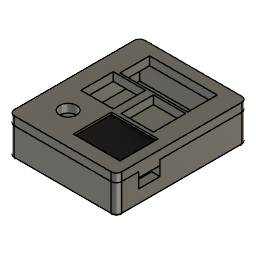
Hackpad case (Autodesk Fusion 360 design; units mm, degrees)
Autodesk Fusion 360 part; units mm, degrees
sketch "Sketch1" plane through (0, 0, 0) normal (0, 0, 1) x (1, 0, 0)
  line L0 (-43.0674, 74.3776) -> (-0.0674, 74.3776)
  line L1 (-0.0674, 74.3776) -> (-0.0674, 20.3776)
  line L2 (-0.0674, 20.3776) -> (-43.0674, 20.3776)
  line L3 (-43.0674, 20.3776) -> (-43.0674, 74.3776)
  line L4 (-0.0674, 20.3776) -> (-0.0674, 28.1436)
  line L5 (-0.0674, 26.9886) -> (3.8652, 26.9886)
  line L6 (-0.0674, 37.0541) -> (3.8652, 37.0541)
  line L7 (-47, 78.3102) -> (3.8652, 78.3102)
  line L8 (3.8652, 78.3102) -> (3.8652, 16.445)
  line L9 (3.8652, 16.445) -> (-47, 16.445)
  line L10 (-47, 16.445) -> (-47, 78.3102)
  dimension "d1" = 54
  dimension "d2" = 43
  constraint horizontal L0
  constraint vertical L1
  constraint horizontal L2
  constraint vertical L3
  constraint coincident L1 L4.end
  constraint coincident L1 L5.start
  constraint perpendicular L1 L5
  constraint coincident L1 L6.start
  constraint perpendicular L1 L6
  constraint horizontal L7
  constraint vertical L8
  constraint horizontal L9
  constraint vertical L10
  constraint coincident L5.end L8
  measures "d1" distance of L0.start L2.end
  measures "d2" distance of L0.start L0.end
extrude "Extrude1" add sketch "Sketch1" along normal blind 4 makes body 1
extrude "Extrude2" add sketch "Sketch1" along normal blind 13 contours L0 L1 L2 L3 L4 L5 L6 L7 L8 L9 L10 | L1 L4 L5 L6 L8 bodies 1
extrude "Extrude3" add sketch "Sketch1" along normal blind 14 contours L0 L1 L2 L3 L4 L5 L6 L7 L8 L9 L10 bodies 1
extrude "Extrude4" cut 1 faces at (2.5543, 33.6989, 13) along direction (0, 0, -1) blind 5 on bodies 1 bodies 1
fillet "Fillet1" radius 2.5 4 edges at (3.8652, 78.3102, 7) (-47, 78.3102, 7) (-47, 16.445, 7) (3.8652, 16.445, 7) on bodies 1
fillet "Fillet2" radius 1 8 edges at (3.1329, 17.1773, 0) (-21.5674, 16.445, 0) (-46.2678, 17.1773, 0) (-47, 47.3776, 0) (-46.2678, 77.578, 0) (-21.5674, 78.3102, 0) (3.1329, 77.578, 0) (3.8652, 47.3776, 0) on bodies 1
sketch "Sketch2" plane through (0, 0, 0) normal (0, 0, -1) x (1, 0, 0)
  arc A0 (2.8652, -18.945) -> (1.3652, -17.445) centre (1.3652, -18.945) ccw
  line L0 (1.3652, -17.445) -> (-44.5, -17.445)
  arc A1 (-44.5, -17.445) -> (-46, -18.945) centre (-44.5, -18.945) ccw
  line L1 (-46, -18.945) -> (-46, -75.8102)
  arc A2 (-46, -75.8102) -> (-44.5, -77.3102) centre (-44.5, -75.8102) ccw
  line L2 (-44.5, -77.3102) -> (1.3652, -77.3102)
  arc A3 (1.3652, -77.3102) -> (2.8652, -75.8102) centre (1.3652, -75.8102) ccw
  line L3 (2.8652, -75.8102) -> (2.8652, -18.945)
  circle A4 centre (-40, -25) radius 2.9748
  circle A5 centre (-31.25, -25) radius 2.9748
  circle A6 centre (-22.5, -25) radius 2.9748
  circle A7 centre (-13.75, -25) radius 2.9748
  circle A8 centre (-5, -25) radius 2.9748
  circle A9 centre (-40, -36.25) radius 2.9748
  circle A10 centre (-31.25, -36.25) radius 2.9748
  circle A11 centre (-22.5, -36.25) radius 2.9748
  circle A12 centre (-13.75, -36.25) radius 2.9748
  circle A13 centre (-5, -36.25) radius 2.9748
  circle A14 centre (-40, -47.5) radius 2.9748
  circle A15 centre (-31.25, -47.5) radius 2.9748
  circle A16 centre (-22.5, -47.5) radius 2.9748
  circle A17 centre (-13.75, -47.5) radius 2.9748
  circle A18 centre (-5, -47.5) radius 2.9748
  circle A19 centre (-40, -58.75) radius 2.9748
  circle A20 centre (-31.25, -58.75) radius 2.9748
  circle A21 centre (-22.5, -58.75) radius 2.9748
  circle A22 centre (-13.75, -58.75) radius 2.9748
  circle A23 centre (-5, -58.75) radius 2.9748
  circle A24 centre (-40, -70) radius 2.9748
  circle A25 centre (-31.25, -70) radius 2.9748
  circle A26 centre (-22.5, -70) radius 2.9748
  circle A27 centre (-13.75, -70) radius 2.9748
  circle A28 centre (-5, -70) radius 2.9748
  point P0 (-33, -25)
  point P1 (-26, -25)
  point P2 (-19, -25)
  point P3 (-12, -25)
  point P4 (-5, -25)
  point P5 (-40, -50)
  point P6 (-33, -50)
  point P7 (-26, -50)
  point P8 (-19, -50)
  point P9 (-12, -50)
  point P10 (-5, -50)
  point P11 (-40, -75)
  point P12 (-33, -75)
  point P13 (-26, -75)
  point P14 (-19, -75)
  point P15 (-12, -75)
  point P16 (-5, -75)
  dimension "d19" = 35
  dimension "d20" = -50
  dimension "d23" = 35
  dimension "d24" = -45
extrude "Extrude5" cut sketch "Sketch2" against normal blind 1 contours A4 | A5 | A6 | A7 | A9 | A10 | A11 | A12 | A13 | A14 | A15 | A16 | A17 | A18 | A19 | A20 | A21 | A22 | A23 | A25 | A26 | A27 | A28 bodies 1
extrude "Extrude6" cut sketch "Sketch2" against normal blind 1 contours A24 bodies 1
extrude "Extrude7" cut sketch "Sketch2" against normal blind 1 contours A8 bodies 1
sketch "Sketch3" plane through (0, 0, 14) normal (0, 0, 1) x (-1, 0, 0)
  arc A0 (-1.3652, -16.445) -> (-3.8652, -18.945) centre (-1.3652, -18.945) ccw
  line L0 (-3.8652, -18.945) -> (-3.8652, -26.9886)
  line L1 (-3.8652, -26.9886) -> (0.0674, -26.9886)
  line L2 (0.0674, -26.9886) -> (0.0674, -20.3776)
  line L3 (0.0674, -20.3776) -> (43.0674, -20.3776)
  line L4 (43.0674, -20.3776) -> (43.0674, -74.3776)
  line L5 (43.0674, -74.3776) -> (0.0674, -74.3776)
  line L6 (0.0674, -74.3776) -> (0.0674, -37.0541)
  line L7 (0.0674, -37.0541) -> (-3.8652, -37.0541)
  line L8 (-3.8652, -37.0541) -> (-3.8652, -75.8102)
  arc A1 (-3.8652, -75.8102) -> (-1.3652, -78.3102) centre (-1.3652, -75.8102) ccw
  line L9 (-1.3652, -78.3102) -> (44.5, -78.3102)
  arc A2 (44.5, -78.3102) -> (47, -75.8102) centre (44.5, -75.8102) ccw
  line L10 (47, -75.8102) -> (47, -18.945)
  arc A3 (47, -18.945) -> (44.5, -16.445) centre (44.5, -18.945) ccw
  line L11 (44.5, -16.445) -> (-1.3652, -16.445)
  line L12 (47.0064, -78.3102) -> (-3.8652, -78.3102)
  line L13 (-3.8652, -78.3102) -> (-3.8652, -16.4024)
  line L14 (-3.8652, -16.4024) -> (47.0064, -16.4024)
  line L15 (47.0064, -16.4024) -> (47.0064, -78.3102)
  constraint horizontal L12
  constraint vertical L13
  constraint horizontal L14
  constraint vertical L15
move_body "Move1" bodies 1 to x (1, 0, 0) y (0, 1, 0) z (0, 0, 1) at (0, -3, 0)
extrude "Extrude8" cut 1 faces at (2.5543, 30.6989, 8) along direction (0, 0, -1) blind 1 on bodies 1 bodies 1
sketch "Sketch4" plane through (0, 23.9886, 0) normal (0, 1, 0) x (-1, 0, 0)
  line L0 (0.0674, 7) -> (0.0674, 14)
  line L1 (0.0674, 14) -> (-3.8652, 14)
  line L2 (-3.8652, 14) -> (-3.8652, 7)
  line L3 (-3.8652, 7) -> (0.0674, 7)
sketch "Sketch5" plane through (0, 0, 14) normal (0, 0, 1) x (-1, 0, 0)
  arc A0 (-1.3652, -13.445) -> (-3.8652, -15.945) centre (-1.3652, -15.945) ccw
  line L0 (-3.8652, -15.945) -> (-3.8652, -23.9886)
  line L1 (-3.8652, -23.9886) -> (0.0674, -23.9886)
  line L2 (0.0674, -23.9886) -> (0.0674, -17.3776)
  line L3 (0.0674, -17.3776) -> (43.0674, -17.3776)
  line L4 (43.0674, -17.3776) -> (43.0674, -71.3776)
  line L5 (43.0674, -71.3776) -> (0.0674, -71.3776)
  line L6 (0.0674, -71.3776) -> (0.0674, -34.0541)
  line L7 (0.0674, -34.0541) -> (-3.8652, -34.0541)
  line L8 (-3.8652, -34.0541) -> (-3.8652, -72.8102)
  arc A1 (-3.8652, -72.8102) -> (-1.3652, -75.3102) centre (-1.3652, -72.8102) ccw
  line L9 (-1.3652, -75.3102) -> (44.5, -75.3102)
  arc A2 (44.5, -75.3102) -> (47, -72.8102) centre (44.5, -72.8102) ccw
  line L10 (47, -72.8102) -> (47, -15.945)
  arc A3 (47, -15.945) -> (44.5, -13.445) centre (44.5, -15.945) ccw
  line L11 (44.5, -13.445) -> (-1.3652, -13.445)
  line L12 (39.119, -54.9533) -> (23.8738, -54.9533)
  line L13 (23.8738, -54.9533) -> (23.8738, -39.7082)
  line L14 (23.8738, -39.7082) -> (39.119, -39.7082)
  line L15 (39.119, -39.7082) -> (39.119, -54.9533)
  line L16 (24.9964, -53.8308) -> (37.9964, -53.8308)
  line L17 (37.9964, -53.8308) -> (37.9964, -40.8308)
  line L18 (37.9964, -40.8308) -> (24.9964, -40.8308)
  line L19 (24.9964, -40.8308) -> (24.9964, -53.8308)
  line L20 (37.9964, -40.8308) -> (39.119, -39.7082)
  line L21 (24.9964, -53.8308) -> (23.8738, -54.9533)
  line L22 (39.119, -54.9533) -> (23.8738, -54.9533)
  line L23 (39.119, -39.7082) -> (39.119, -54.9533)
  line L24 (37.9964, -40.8308) -> (24.9964, -40.8308)
  line L25 (23.8738, -39.7082) -> (39.119, -39.7082)
  line L26 (37.9964, -40.8308) -> (39.119, -39.7082)
  line L27 (37.9964, -53.8308) -> (37.9964, -40.8308)
  line L28 (24.9964, -53.8308) -> (37.9964, -53.8308)
  line L29 (23.8738, -54.9533) -> (23.8738, -39.7082)
  line L30 (24.9964, -40.8308) -> (24.9964, -53.8308)
  line L31 (24.9964, -53.8308) -> (23.8738, -54.9533)
  line L32 (4.8738, -39.7082) -> (20.119, -39.7082)
  line L33 (4.8738, -54.9533) -> (4.8738, -39.7082)
  line L34 (5.9964, -53.8308) -> (18.9964, -53.8308)
  line L35 (5.9964, -40.8308) -> (5.9964, -53.8308)
  line L36 (18.9964, -40.8308) -> (5.9964, -40.8308)
  line L37 (20.119, -39.7082) -> (20.119, -54.9533)
  line L38 (20.119, -54.9533) -> (4.8738, -54.9533)
  line L39 (5.9964, -40.8308) -> (5.9964, -53.8308)
  line L40 (4.8738, -39.7082) -> (20.119, -39.7082)
  line L41 (20.119, -54.9533) -> (4.8738, -54.9533)
  line L42 (18.9964, -40.8308) -> (5.9964, -40.8308)
  line L43 (5.9964, -53.8308) -> (18.9964, -53.8308)
  line L44 (5.9964, -53.8308) -> (4.8738, -54.9533)
  line L45 (18.9964, -53.8308) -> (18.9964, -40.8308)
  line L46 (18.9964, -53.8308) -> (18.9964, -40.8308)
  line L47 (5.9964, -53.8308) -> (4.8738, -54.9533)
  line L48 (4.8738, -54.9533) -> (4.8738, -39.7082)
  line L49 (18.9964, -40.8308) -> (20.119, -39.7082)
  line L50 (18.9964, -40.8308) -> (20.119, -39.7082)
  line L51 (20.119, -39.7082) -> (20.119, -54.9533)
  line L52 (37, -70) -> (5, -70)
  line L53 (5, -70) -> (5, -56)
  line L54 (5, -56) -> (37, -56)
  line L55 (37, -56) -> (37, -70)
  line L56 (34, -32.5) -> (34, -24.5)
  circle A4 centre (34, -28.5) radius 4
  line L57 (23, -38) -> (1, -38)
  line L58 (1, -38) -> (1, -20.0095)
  line L59 (1, -20.0095) -> (23, -20.0095)
  line L60 (23, -20.0095) -> (23, -38)
  line L61 (-3.8652, -75.6763) -> (-3.8652, -13.0993)
  line L62 (-3.8652, -13.0993) -> (47, -13.0993)
  line L63 (47, -13.0993) -> (47, -75.6763)
  dimension "d33" = 13
  dimension "d34" = 13
  dimension "d35" = 13
  dimension "d36" = 13
  constraint horizontal L12
  constraint vertical L13
  constraint horizontal L14
  constraint vertical L15
  constraint horizontal L16
  constraint vertical L17
  constraint horizontal L18
  constraint vertical L19
  constraint equal L16 L19
  constraint equal L20 L21
  constraint parallel L20 L21
  constraint equal L12 L15
  constraint horizontal L22
  constraint vertical L29
  constraint horizontal L25
  constraint vertical L23
  constraint horizontal L28
  constraint vertical L27
  constraint horizontal L24
  constraint vertical L30
  constraint equal L28 L30
  constraint equal L26 L31
  constraint parallel L26 L31
  constraint equal L22 L23
  constraint horizontal L41
  constraint vertical L33
  constraint horizontal L40
  constraint vertical L37
  constraint horizontal L43
  constraint vertical L46
  constraint horizontal L36
  constraint vertical L35
  constraint equal L35 L43
  constraint equal L44 L50
  constraint parallel L44 L50
  constraint equal L37 L41
  constraint horizontal L38
  constraint vertical L48
  constraint horizontal L32
  constraint vertical L51
  constraint horizontal L34
  constraint vertical L45
  constraint horizontal L42
  constraint vertical L39
  constraint equal L34 L39
  constraint equal L47 L49
  constraint parallel L47 L49
  constraint equal L38 L51
  constraint horizontal L52
  constraint vertical L53
  constraint horizontal L54
  constraint vertical L55
  constraint vertical L56
  constraint horizontal L57
  constraint vertical L58
  constraint horizontal L59
  constraint vertical L60
  constraint vertical L61
  constraint horizontal L62
  constraint vertical L63
  measures "d33" distance of L16.end L17.end
  measures "d34" distance of L17.end L16.end
  measures "d35" distance of L36.start L34.end
  measures "d36" distance of L36.start L34.end
extrude "Extrude1'" add sketch "Sketch5" along normal blind 4 separate body contours A0 L0 L1 L2 L3 L4 L5 L6 L7 L8 A1 L9 A2 L10 A3 L11 L61 L63 | L1 L2 L3 L4 L5 L6 L7 L61 makes body 2 in component "Component"
sketch "Sketch6" plane through (0, 0, 14) normal (0, 0, -1) x (1, 0, 0)
  line L0 (-20.119, -39.7082) -> (-4.8738, -39.7082)
  line L1 (-4.8738, -39.7082) -> (-4.8738, -54.9533)
  line L2 (-4.8738, -54.9533) -> (-20.119, -54.9533)
  line L3 (-20.119, -54.9533) -> (-20.119, -39.7082)
  line L4 (-23.8738, -54.9533) -> (-39.119, -54.9533)
  line L5 (-39.119, -54.9533) -> (-39.119, -39.7082)
  line L6 (-39.119, -39.7082) -> (-23.8738, -39.7082)
  line L7 (-23.8738, -39.7082) -> (-23.8738, -54.9533)
  circle A0 centre (-34, -28.5) radius 4
  line L8 (-37, -56) -> (-5, -56)
  line L9 (-5, -56) -> (-5, -70)
  line L10 (-5, -70) -> (-37, -70)
  line L11 (-37, -70) -> (-37, -56)
  line L12 (-23, -20.0095) -> (-1, -20.0095)
  line L13 (-1, -20.0095) -> (-1, -38)
  line L14 (-1, -38) -> (-23, -38)
  line L15 (-23, -38) -> (-23, -20.0095)
  arc A1 (1.3652, -75.3102) -> (3.8652, -72.8102) centre (1.3652, -72.8102) ccw
  line L16 (3.8652, -72.8102) -> (3.8652, -15.945)
  arc A2 (3.8652, -15.945) -> (1.3652, -13.445) centre (1.3652, -15.945) ccw
  line L17 (1.3652, -13.445) -> (-44.5, -13.445)
  arc A3 (-44.5, -13.445) -> (-47, -15.945) centre (-44.5, -15.945) ccw
  line L18 (-47, -15.945) -> (-47, -72.8102)
  arc A4 (-47, -72.8102) -> (-44.5, -75.3102) centre (-44.5, -72.8102) ccw
  line L19 (-44.5, -75.3102) -> (1.3652, -75.3102)
  line L20 (3.8652, -15.945) -> (3.8652, -24)
  line L21 (3.8652, -24) -> (-1, -24)
  line L22 (-1, -24) -> (-1, -34.049)
  line L23 (-1, -34.049) -> (3.8652, -34.049)
  line L24 (3.8652, -34.049) -> (3.8652, -24)
  constraint coincident L16.end A2.start
  constraint coincident L16 L20.end
  constraint horizontal L21
  constraint vertical L22
  constraint horizontal L23
  constraint vertical L24
  constraint coincident L13 L22.end
extrude "Extrude2'" add sketch "Sketch6" along normal blind 2.5 contours L13 L16 L21 L22 L23 L24 bodies 2 in component "Component"
sketch "Sketch7" plane through (-23, 0, 0) normal (1, 0, 0) x (0, 1, 0)
  line L0 (20.0095, 14) -> (38, 14)
  line L1 (38, 14) -> (38, 18)
  line L2 (38, 18) -> (20.0095, 18)
  line L3 (20.0095, 18) -> (20.0095, 14)
  line L4 (20.0095, 14) -> (38, 14)
  line L5 (38, 14) -> (38, 17)
  line L6 (38, 17) -> (20.0095, 17)
  line L7 (20.0095, 17) -> (20.0095, 14)
  constraint horizontal L4
  constraint vertical L5
  constraint horizontal L6
  constraint vertical L7
  constraint coincident L1 L5.end
  constraint coincident L0.start L3.end
extrude "Extrude3'" add sketch "Sketch7" along normal blind 22 contours L0 L1 L3 L4 L5 L6 L7 bodies 2 in component "Component"
component "Component" placed x (1, 0, 0) y (0, 1, 0) z (0, 0, 1) at (0, 0, 0)
